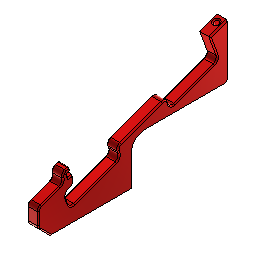
PCB bracket v5 (Autodesk Fusion 360 design; units mm, degrees)
Autodesk Fusion 360 part; units mm, degrees
sketch "Esquisse1" plane through (0, 0, 0) normal (1, 0, 0) x (0, 1, 0)
  line L0 (0, 0) -> (0, 15) construction
  line L1 (30, 0) -> (30, 15) construction
  line L2 (32.5, 0) -> (32.5, 13)
  line L3 (32.5, 13) -> (38.5, 19)
  line L4 (38.5, 19) -> (73.7, 19)
  line L5 (32.5, 0) -> (-2.5, 0)
  line L6 (-2.5, 0) -> (-8, 5.5)
  line L7 (-8, 13) -> (73.0506, 42.5)
  line L8 (14.3198, 21.1237) -> (18.082, 10.7871) construction
  line L9 (70.7014, 41.6449) -> (74.4636, 31.3083) construction
  line L10 (46.2693, 32.7524) -> (50.0316, 22.4158) construction
  line L11 (11.9706, 20.2687) -> (15.7328, 9.9321) construction
  line L12 (15.7328, 9.9321) -> (18.082, 10.7871) construction
  line L13 (73.0506, 42.5) -> (76.8128, 32.1634) construction
  line L14 (76.8128, 32.1634) -> (74.4636, 31.3083) construction
  line L15 (3.1375, 17.0537) -> (1.8378, 20.6245)
  line L16 (1.8378, 20.6245) -> (5.2207, 21.8558)
  line L17 (5.2207, 21.8558) -> (5.9047, 19.9764)
  line L18 (5.9047, 19.9764) -> (4.4012, 19.4292)
  line L19 (4.4012, 19.4292) -> (5.0168, 17.7377)
  line L20 (-2.5, 0) -> (-2.5, 15) construction
  line L21 (-2.5, 15) -> (2.5, 15) construction
  line L22 (2.5, 15) -> (2.5, 0) construction
  line L23 (32.5, 0) -> (32.5, 15) construction
  line L24 (32.5, 15) -> (27.5, 15) construction
  line L25 (27.5, 15) -> (27.5, 0) construction
  line L26 (-8, 5.5) -> (-8, 13)
  line L27 (73.7, 19) -> (73.7, 40.7157)
  line L28 (73.0506, 42.5) -> (73.7, 40.7157)
  dimension "d1" = 30
  dimension "d2" = 15
  dimension "d3" = 2.5
  dimension "d4" = 2.5
  dimension "d5" = 19
  dimension "d6" = 135
  dimension "d7" = 13
  dimension "d8" = 60
  dimension "d9" = 26
  dimension "d10" = 11
  dimension "d11" = 2.5
  dimension "d12" = 2.5
  dimension "d14" = 3.6
  dimension "d15" = 3.8
  dimension "d16" = 2
  dimension "d17" = 2
  dimension "d18" = 5.5
  dimension "d19" = 13
  dimension "d20" = 135
  dimension "d21" = 81.7
  dimension "d23" = 42.5
  dimension "d24" = 110
  dimension "d25" = 74.4
  constraint coincident L0.start origin
  constraint vertical L0
  constraint vertical L1
  constraint horizontal L0.start L1.start
  constraint equal L0 L1
  constraint parallel L1 L2
  constraint perpendicular L2 L4
  constraint perpendicular L1 L5
  constraint coincident L0.start L5
  constraint coincident L7 L8.start
  constraint perpendicular L7 L8
  constraint coincident L7 L9.start
  constraint perpendicular L7 L9
  constraint coincident L7 L10.start
  constraint perpendicular L7 L10
  constraint equal L8 L10
  constraint equal L9 L10
  constraint coincident L7 L11.start
  constraint perpendicular L7 L11
  constraint coincident L7 L13.start
  constraint perpendicular L7 L13
  constraint perpendicular L13 L14
  constraint perpendicular L11 L12
  constraint coincident L7.end L13.start
  constraint coincident L7 L15.start
  constraint perpendicular L7 L15
  constraint perpendicular L15 L16
  constraint perpendicular L16 L17
  constraint perpendicular L17 L18
  constraint coincident L7 L19.end
  constraint perpendicular L7 L19
  constraint perpendicular L5 L20
  constraint perpendicular L20 L21
  constraint coincident L5 L22.end
  constraint perpendicular L5 L22
  constraint midpoint L0.end L21
  constraint perpendicular L5 L23
  constraint perpendicular L2 L24
  constraint coincident L5 L25.end
  constraint perpendicular L5 L25
  constraint midpoint L1.end L24
  constraint vertical L26
  constraint coincident L7.start L26.end
  constraint coincident L13 L27.end
  constraint perpendicular L4 L27
  measures "d1" distance of L0 L1
  measures "d2" distance of L1.start L1.end
  measures "d3" distance of L1 L2
  measures "d4" distance of L0.start L5.end
  measures "d5" distance of L1.start L4
  measures "d6" angle of L3 L4
  measures "d7" distance of L2.start L2.end
  measures "d8" distance of L8 L9
  measures "d9" distance of L9 L10
  measures "d10" distance of L8.start L8.end
  measures "d11" distance of L8 L11
  measures "d12" distance of L9 L13
  measures "d14" distance of L15.end L16.end
  measures "d15" distance of L7 L16
  measures "d16" distance of L15 L19
  measures "d17" distance of L16.end L17.end
  measures "d18" distance of L20 L26
  measures "d19" vertical distance of L5.end L7.start
  measures "d20" angle of L6 L26
  measures "d21" distance of L4.end L26
  measures "d23" vertical distance of L1.start L7.end
  measures "d24" angle of L7 L26
  measures "d25" distance of L7.end L15.start
sketch "Esquisse2" plane through (0, 0, 0) normal (1, 0, 0) x (0, 1, 0)
  line L0 (-8, 13) -> (6.5652, 18.3013)
  line L1 (6.5652, 18.3013) -> (8.2753, 13.6028)
  line L2 (8.2753, 13.6028) -> (67.2431, 35.0654)
  line L3 (67.2431, 35.0654) -> (65.533, 39.7638)
  line L4 (65.533, 39.7638) -> (73.0506, 42.5)
  line L5 (73.0506, 42.5) -> (73.7, 40.7157)
  line L6 (73.7, 40.7157) -> (73.7, 19)
  line L7 (73.7, 19) -> (38.5, 19)
  line L8 (-8, 13) -> (73.0506, 42.5) construction
  line L9 (38.5, 19) -> (32.5, 14) construction
  line L10 (32.5, 14) -> (32.5, 0)
  line L11 (32.5, 0) -> (-2.5, 0)
  line L12 (-2.5, 0) -> (-8, 5.5)
  line L13 (-8, 5.5) -> (-8, 13)
  line L14 (5.2207, 21.8558) -> (5.9047, 19.9764)
  line L15 (1.8378, 20.6245) -> (5.2207, 21.8558)
  line L16 (5.9047, 19.9764) -> (4.4012, 19.4292)
  line L17 (4.4012, 19.4292) -> (5.0168, 17.7377)
  line L18 (3.1375, 17.0537) -> (1.8378, 20.6245)
  spline S0 degree 5 poles (38.5, 19) (38.054, 19) (37.2045, 18.9542) (36.0574, 18.7481) (34.7618, 18.2262) (33.5048, 17.2265) (32.8287, 16.1486) (32.5598, 15.1546) (32.5, 14.4002) (32.5, 14) knots 0 0 0 0 0 0 0.2 0.4 0.6 0.8 1 1 1 1 1 1
  line L19 (39.441, 19) -> (37.559, 19)
  line L20 (32.5, 14.7985) -> (32.5, 13.2015)
  circle A0 centre (17.6723, 17.0231) radius 3.5
  circle A1 centre (55.26, 30.7039) radius 3.5
  line L21 (8.2753, 13.6028) -> (10.3275, 7.9647)
  line L22 (10.3275, 7.9647) -> (27.2419, 14.1211)
  line L23 (27.2419, 14.1211) -> (25.1898, 19.7592)
  line L24 (25.5318, 18.8195) -> (46.9119, 26.6012)
  line L25 (46.9119, 26.6012) -> (48.622, 21.9028)
  line L26 (48.622, 21.9028) -> (69.2953, 29.4272)
  line L27 (69.2953, 29.4272) -> (67.2431, 35.0654)
  point P0 (-8, 13)
  point P1 (73.0506, 42.5)
  point P2 (73.7, 19)
  point P3 (-8, 5.5)
  point P4 (32.5, 0)
  point P5 (38.5, 19)
  point P6 (-2.5, 0)
  dimension "d26" = 15.5
  dimension "d27" = 5
  dimension "d28" = 8
  dimension "d49" = 14
  dimension "d53" = 7
  dimension "d54" = 10
  dimension "d55" = 40
  dimension "d57" = 6
  dimension "d58" = 18
  dimension "d60" = 22
  dimension "d61" = 1
  constraint perpendicular L0 L1
  constraint perpendicular L1 L2
  constraint perpendicular L0 L3
  constraint perpendicular L3 L4
  constraint perpendicular L4 L5
  constraint vertical L6
  constraint perpendicular L6 L7
  constraint coincident P0 L0.start
  constraint collinear L0 L8
  constraint collinear L0 L4
  constraint coincident P1 L4.end
  constraint coincident P2 L6.end
  constraint perpendicular L7 L10
  constraint perpendicular L10 L11
  constraint coincident P3 L12.end
  constraint coincident P4 L10.end
  constraint coincident P5 L7.end
  constraint coincident L10 L9.end
  constraint coincident L9.end L10.start
  constraint coincident P6 L11.end
  constraint midpoint P5 L19
  constraint midpoint L9.end L20
  constraint coincident L10 L20.end
  constraint collinear L7 L19
  constraint coincident L2 A0.centre
  constraint coincident L2 A1.centre
  constraint equal A0 A1
  constraint coincident L2 L1.end
  constraint perpendicular L2 L21
  constraint perpendicular L21 L22
  constraint coincident L2 L23.end
  constraint perpendicular L2 L23
  constraint coincident L23 L24.start
  constraint perpendicular L24 L25
  constraint perpendicular L23 L26
  constraint coincident L2 L3.start
  constraint perpendicular L2 L27
  constraint perpendicular L23 L24
  constraint collinear L22 L26
  constraint collinear L1 L21
  constraint collinear L3 L27
  measures "d26" distance of P0 L0.end
  measures "d27" distance of L0.end L1.end
  measures "d28" distance of L3.end P1
  measures "d49" distance of L9.end P4
  measures "d53" diameter of A0
  measures "d54" distance of L1.end A0.centre
  measures "d55" distance of A0.centre A1.centre
  measures "d57" distance of L1.end L21.end
  measures "d58" distance of L21.end L22.end
  measures "d60" distance of L25.end L26.end
  measures "d61" distance of L2 L24
extrude "Extrusion1" add sketch "Esquisse2" sketch "Esquisse1" along normal mid plane 4.8 contours L0 L1 L3 L4 L5 L6 L7 L10 L11 L12 L13 S0 L19 L20 L21 L22 L23 L24 L25 L26 L27 of sketch 2 contours L7 L15 L16 L17 L18 L19
fillet "Congé1" radius 2 1 edges at (0, 1.8378, 20.6245)
fillet "Congé1" radius 0.5 2 edges at (0, 5.2207, 21.8558) (0, 5.9047, 19.9764)
sketch "Esquisse4" plane through (0, 0, 0) normal (0, 0, -1) x (1, 0, 0)
  line L0 (-2.4, -32.5) -> (2.4, -32.5)
  line L1 (2.4, -32.5) -> (2.4, 2.5)
  line L2 (2.4, 2.5) -> (-2.4, 2.5)
  line L3 (-2.4, 2.5) -> (-2.4, -32.5)
  point P0 (0, -30)
  point P1 (0, -30)
  constraint coincident P1 P0
hole "Perçage1" at (0, 0, 0) at (0, 30, 0) direction (0, 0, 1) diameter 2 depth 10 tip angle 118 countersink diameter 3 countersink angle 90
sketch "Esquisse5" plane through (0, -5.1139, 14.0504) normal (0, -0.34202, 0.939693) x (1, 0, 0)
  line L0 (-2.4, 75.181) -> (2.4, 75.181)
  line L1 (2.4, 75.181) -> (2.4, 83.181)
  line L2 (2.4, 83.181) -> (-2.4, 83.181)
  line L3 (-2.4, 83.181) -> (-2.4, 75.181)
  point P0 (0, 80.681)
  point P1 (0, 80.681)
  constraint coincident P1 P0
hole "Perçage2" at (0, 70.7014, 41.6449) direction (0, 0.34202, -0.939693) diameter 2 depth 5 tip angle 118 countersink diameter 3 countersink angle 90
sketch "Esquisse6" plane through (2.4, 0, 0) normal (1, 0, 0) x (0, 1, 0)
  arc A0 (5.4349, 19.8054) -> (5.7337, 20.4463) centre (5.2639, 20.2753) ccw
  line L0 (5.7337, 20.4463) -> (5.3917, 21.386)
  arc A1 (5.3917, 21.386) -> (4.7508, 21.6848) centre (4.9218, 21.2149) ccw
  line L1 (4.7508, 21.6848) -> (3.7172, 21.3086)
  arc A2 (3.7172, 21.3086) -> (2.5218, 18.7451) centre (4.4012, 19.4292) ccw
  line L2 (2.5218, 18.7451) -> (3.1375, 17.0537)
  line L3 (3.1375, 17.0537) -> (-8, 13)
  line L4 (-8, 13) -> (-8, 5.5)
  line L5 (-8, 5.5) -> (-2.5, 0)
  line L6 (-2.5, 0) -> (32.5, 0)
  line L7 (32.5, 0) -> (32.5, 14)
  spline S0 degree 5 poles (32.5, 14) (32.5, 14.4002) (32.5598, 15.1546) (32.8287, 16.1486) (33.5048, 17.2265) (34.7618, 18.2262) (36.0574, 18.7481) (37.2045, 18.9542) (38.054, 19) (38.5, 19) knots -1 -1 -1 -1 -1 -1 -0.8 -0.6 -0.4 -0.2 0 0 0 0 0 0
  line L8 (38.5, 19) -> (73.7, 19)
  line L9 (73.7, 19) -> (73.7, 40.7157)
  line L10 (73.7, 40.7157) -> (73.0506, 42.5)
  line L11 (73.0506, 42.5) -> (65.533, 39.7638)
  line L12 (65.533, 39.7638) -> (69.2953, 29.4272)
  line L13 (69.2953, 29.4272) -> (48.622, 21.9028)
  line L14 (48.622, 21.9028) -> (46.9119, 26.6012)
  line L15 (46.9119, 26.6012) -> (25.5318, 18.8195)
  line L16 (25.5318, 18.8195) -> (27.2419, 14.1211)
  line L17 (27.2419, 14.1211) -> (10.3275, 7.9647)
  line L18 (10.3275, 7.9647) -> (6.5652, 18.3013)
  line L19 (6.5652, 18.3013) -> (5.0168, 17.7377)
  line L20 (5.0168, 17.7377) -> (4.4012, 19.4292)
  line L21 (4.4012, 19.4292) -> (5.4349, 19.8054)
  line L22 (10.3275, 7.9647) -> (5.629, 6.2546)
  line L23 (5.629, 6.2546) -> (3.2349, 12.8324)
  line L24 (3.2349, 12.8324) -> (7.9333, 14.5425)
  dimension "d62" = 7
  dimension "d63" = 5
  constraint coincident L17.end L18.start
  constraint perpendicular L18 L22
  constraint perpendicular L17 L23
  constraint coincident L18 L24.end
  constraint perpendicular L18 L24
  measures "d62" distance of L22.end L23.end
  measures "d63" distance of L17.end L22.end
extrude "Extrusion2" cut sketch "Esquisse6" against normal up to surface (4.8 mm away) contours L18 L22 L23 L24
fillet "Congé2" radius 2 13 edges at (0, 73.7, 40.7157) (0, -8, 13) (0, 73.7, 19) (0, -8, 5.5) (0, 3.1375, 17.0537) (0, 27.2419, 14.1211) (0, 25.5318, 18.8195) (0, 46.9119, 26.6012) (0, 48.622, 21.9028) (0, 69.2953, 29.4272) (0, 5.629, 6.2546) (0, 3.2349, 12.8324) (0, 7.9333, 14.5425)
chamfer "Chanfrein1" distance 0.5 angle 45 2 faces at (2.4, 21.7903, 6.7919) (-2.4, 21.7903, 6.7919)
equation "d4 = d3"
equation "d17 = d16"
named bodies: "PCB Bracket"
